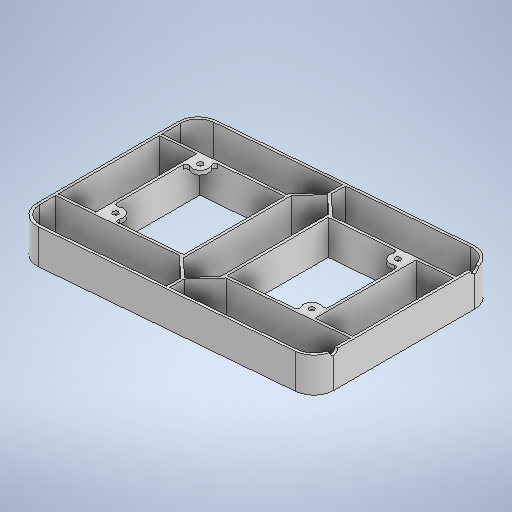
# Autodesk Inventor part: Divider
Saved by Autodesk Inventor 2025.2 (Build 292293000, 293)
## iProperties
Created: 2026-02-06
Part Number: Divider
Material: Generic
Document SubType Name: Modeling
Designer: Joefi
Density: 1 g/cm^3
Appearance: Default
Mass: 74.6343 g
Surface Area: 795.136 cm^2
Volume: 74.6343 cm^3
Author: Joefi
Autodesk Inventor part; units mm, degrees
ref_plane "YZ Plane" through (0, 0, 0) normal (1, 0, 0) x (0, 1, 0)
ref_plane "XZ Plane" through (0, 0, 0) normal (0, 1, 0) x (-1, 0, 0)
ref_plane "XY Plane" through (0, 0, 0) normal (0, 0, 1) x (1, 0, 0)
sketch "Sketch2" plane through (0, 0, 0) normal (0, 1, 0) x (-1, 0, 0)
  line L0 (-103.6195, 45.2048) -> (-103.6195, -60.7112)
  arc A0 (-103.6195, -60.7112) -> (-87.3121, -75.6541) centre (-88.6195, -60.7112) ccw
  line L1 (-87.3121, -75.6541) -> (89.9268, -60.1477)
  arc A1 (89.9268, -60.1477) -> (103.6195, -45.2048) centre (88.6195, -45.2048) ccw
  line L2 (103.6195, -45.2048) -> (103.6195, 60.7112)
  arc A2 (103.6195, 60.7112) -> (87.3121, 75.6541) centre (88.6195, 60.7112) ccw
  line L3 (87.3121, 75.6541) -> (-89.9268, 60.1477)
  arc A3 (-89.9268, 60.1477) -> (-103.6195, 45.2048) centre (-88.6195, 45.2048) ccw
  line L4 (-15, -39.213) -> (-73.7032, -44.3489)
  line L5 (-73.7032, -44.3489) -> (-73.7032, 31.4525)
  line L6 (-73.7032, 31.4525) -> (-15, 36.5884)
  line L7 (-15, 36.5884) -> (-15, -39.213)
  line L8 (73.7032, 44.3489) -> (73.7032, -31.4525)
  line L9 (73.7032, -31.4525) -> (15, -36.5884)
  line L10 (15, -36.5884) -> (15, 39.213)
  line L11 (15, 39.213) -> (73.7032, 44.3489)
  line L12 (-75.7032, -44.5239) -> (-101.6195, -46.7912)
  line L13 (-101.6195, -46.7912) -> (-101.6195, 29.0101)
  line L14 (-101.6195, 29.0101) -> (-75.7032, 31.2775)
  line L15 (-75.7032, 31.2775) -> (-75.7032, -44.5239)
  line L16 (16.0813, -38.5014) -> (101.6195, -31.0178)
  line L17 (101.6195, -31.0178) -> (101.6195, -45.2048)
  arc A4 (89.7525, -58.1553) -> (101.6195, -45.2048) centre (88.6195, -45.2048) ccw
  line L18 (89.7525, -58.1553) -> (1, -65.9202)
  line L19 (1, -65.9202) -> (1, -54.9598)
  line L20 (1, -54.9598) -> (16.0813, -38.5014)
  line L21 (-1, -55.3824) -> (-1, -66.0951)
  line L22 (-1, -66.0951) -> (-87.4864, -73.6617)
  arc A5 (-101.6195, -60.7112) -> (-87.4864, -73.6617) centre (-88.6195, -60.7112) ccw
  line L23 (-101.6195, -60.7112) -> (-101.6195, -48.7989)
  line L24 (-101.6195, -48.7989) -> (-16.3281, -41.3368)
  line L25 (-16.3281, -41.3368) -> (-1, -55.3824)
  line L26 (-16.0813, 38.5014) -> (-101.6195, 31.0178)
  line L27 (-101.6195, 31.0178) -> (-101.6195, 45.2048)
  arc A6 (-89.7525, 58.1553) -> (-101.6195, 45.2048) centre (-88.6195, 45.2048) ccw
  line L28 (-89.7525, 58.1553) -> (-1, 65.9202)
  line L29 (-1, 65.9202) -> (-1, 54.9598)
  line L30 (-1, 54.9598) -> (-16.0813, 38.5014)
  line L31 (13, -39.6468) -> (0.1234, -53.6991)
  line L32 (0.1234, -53.6991) -> (-13, -41.6738)
  line L33 (-13, -41.6738) -> (-13, 39.6468)
  line L34 (-13, 39.6468) -> (-0.1234, 53.6991)
  line L35 (-0.1234, 53.6991) -> (13, 41.6738)
  line L36 (13, 41.6738) -> (13, -39.6468)
  line L37 (101.6195, 46.7912) -> (101.6195, -29.0101)
  line L38 (101.6195, -29.0101) -> (75.7032, -31.2775)
  line L39 (75.7032, -31.2775) -> (75.7032, 44.5239)
  line L40 (75.7032, 44.5239) -> (101.6195, 46.7912)
  line L41 (16.3281, 41.3368) -> (1, 55.3824)
  line L42 (1, 55.3824) -> (1, 66.0951)
  line L43 (1, 66.0951) -> (87.4864, 73.6617)
  arc A7 (101.6195, 60.7112) -> (87.4864, 73.6617) centre (88.6195, 60.7112) ccw
  line L44 (101.6195, 60.7112) -> (101.6195, 48.7989)
  line L45 (101.6195, 48.7989) -> (16.3281, 41.3368)
  point P0 (0, 0)
  point P1 (0, 0)
  constraints: 92 end point, 16 point on circle, 8 centre point
extrude "Extrusion1" add sketch "Sketch2" along normal blind 26
sketch "Sketch3" plane through (0, 0, 0) normal (0, -1, 0) x (1, 0, 0)
  line L0 (-15, 39.213) -> (-73.7032, 44.3489) projected
  line L1 (-73.7032, -31.4525) -> (-15, -36.5884) projected
  line L2 (-73.7032, 44.3489) -> (-73.7032, -31.4525) projected
  line L3 (73.7032, 31.4525) -> (15, 36.5884) projected
  line L4 (73.7032, -44.3489) -> (73.7032, 31.4525) projected
  line L5 (15, -39.213) -> (73.7032, -44.3489) projected
  line L6 (-13.5, 41.8938) -> (0.1542, 54.4056) construction
  line L7 (-0.5, 55.1624) -> (-16.1525, 40.8196) construction
  line L8 (-0.5, 66.5533) -> (-0.5, 55.1624) construction
  line L9 (-15, 39.213) -> (-73.7032, 44.3489) construction
  line L10 (-0.1542, -54.4056) -> (-13.5, -39.8412) construction
  line L11 (-16.1525, 40.8196) -> (-102.1195, 48.3407) construction
  line L12 (-102.1195, 48.3407) -> (-102.1195, 60.7112) construction
  line L13 (16.1525, -40.8196) -> (102.1195, -48.3407) construction
  line L14 (102.1195, 45.2048) -> (102.1195, 30.4721) construction
  line L15 (14.5, 37.134) -> (74.2032, 31.9107) construction
  arc A0 (-87.4429, 74.1598) -> (-102.1195, 60.7112) centre (-88.6195, 60.7112) ccw construction
  line L16 (15.8441, 38.0202) -> (0.5, 54.7653) construction
  line L17 (14.5, -39.6712) -> (14.5, 37.134) construction
  line L18 (13.5, 39.8412) -> (13.5, -41.8938) construction
  line L19 (0.5, -66.5533) -> (0.5, -55.1624) construction
  line L20 (0.5, 66.4658) -> (89.7961, 58.6534) construction
  line L21 (102.1195, 30.4721) -> (15.8441, 38.0202) construction
  line L22 (75.2032, 31.8232) -> (102.1195, 29.4683) construction
  line L23 (74.2032, -44.8945) -> (14.5, -39.6712) construction
  line L24 (0.1542, 54.4056) -> (13.5, 39.8412) construction
  line L25 (13.5, -41.8938) -> (-0.1542, -54.4056) construction
  line L26 (-0.5, -54.7653) -> (-0.5, -66.4658) construction
  line L27 (0.5, 54.7653) -> (0.5, 66.4658) construction
  line L28 (-89.8832, -59.6496) -> (87.3557, -75.156) construction
  line L29 (89.8832, 59.6496) -> (-87.3557, 75.156) construction
  line L30 (-87.4429, 74.1598) -> (-0.5, 66.5533) construction
  arc A1 (-87.3557, 75.156) -> (-103.1195, 60.7112) centre (-88.6195, 60.7112) ccw construction
  line L31 (87.4429, -74.1598) -> (0.5, -66.5533) construction
  line L32 (74.2032, 31.9107) -> (74.2032, -44.8945) construction
  line L33 (75.2032, -44.982) -> (75.2032, 31.8232) construction
  line L34 (102.1195, 29.4683) -> (102.1195, -47.3369) construction
  line L35 (102.1195, -48.3407) -> (102.1195, -60.7112) construction
  line L36 (103.1195, -60.7112) -> (103.1195, 45.2048) construction
  arc A2 (-102.1195, -45.2048) -> (-89.7961, -58.6534) centre (-88.6195, -45.2048) ccw construction
  arc A3 (-103.1195, -45.2048) -> (-89.8832, -59.6496) centre (-88.6195, -45.2048) ccw construction
  line L37 (0.5, -55.1624) -> (16.1525, -40.8196) construction
  arc A4 (102.1195, 45.2048) -> (89.7961, 58.6534) centre (88.6195, 45.2048) ccw construction
  arc A5 (103.1195, 45.2048) -> (89.8832, 59.6496) centre (88.6195, 45.2048) ccw construction
  line L38 (-15.8441, -38.0202) -> (-0.5, -54.7653) construction
  line L39 (-0.5, -66.4658) -> (-89.7961, -58.6534) construction
  line L40 (-13.5, -39.8412) -> (-13.5, 41.8938) construction
  line L41 (-15, -36.5884) -> (-15, 39.213) construction
  line L42 (-102.1195, 47.3369) -> (-75.2032, 44.982) construction
  line L43 (-75.2032, 44.982) -> (-75.2032, -31.8232) construction
  line L44 (-73.7032, 44.3489) -> (-73.7032, -31.4525) construction
  line L45 (-102.1195, -29.4683) -> (-102.1195, 47.3369) construction
  line L46 (-75.2032, -31.8232) -> (-102.1195, -29.4683) construction
  line L47 (-103.1195, 60.7112) -> (-103.1195, -45.2048) construction
  line L48 (-73.7032, -31.4525) -> (-15, -36.5884) construction
  line L49 (-102.1195, -45.2048) -> (-102.1195, -30.4721) construction
  line L50 (-102.1195, -30.4721) -> (-15.8441, -38.0202) construction
  line L51 (102.1195, -47.3369) -> (75.2032, -44.982) construction
  arc A6 (87.4429, -74.1598) -> (102.1195, -60.7112) centre (88.6195, -60.7112) ccw construction
  arc A7 (87.3557, -75.156) -> (103.1195, -60.7112) centre (88.6195, -60.7112) ccw construction
  circle A8 centre (-67.7032, -25.9545) radius 6
  circle A9 centre (-67.7032, 37.801) radius 6
  circle A10 centre (68.2032, -38.3467) radius 6
  circle A11 centre (68.2032, 26.4127) radius 6
  circle A12 centre (-67.7032, -25.9545) radius 1.45 construction
  circle A13 centre (-67.7032, 37.801) radius 1.45 construction
  circle A14 centre (68.2032, 26.4127) radius 1.45 construction
  circle A15 centre (68.2032, -38.3467) radius 1.45 construction
  line L52 (-100.0356, -54.4397) -> (-99.164, -44.4778)
  line L53 (-99.164, -44.4778) -> (-95.4115, -44.8061)
  line L54 (-95.4115, -44.8061) -> (-95.4115, 61.1557)
  line L55 (-95.4115, 61.1557) -> (-100.0356, 61.5603)
  line L56 (-100.0356, 61.5603) -> (-99.164, 71.5222)
  line L57 (-99.164, 71.5222) -> (96.0902, 54.4397)
  line L58 (96.0902, 54.4397) -> (95.2186, 44.4778)
  line L59 (95.2186, 44.4778) -> (91.4661, 44.8061)
  line L60 (91.4661, 44.8061) -> (91.4661, -61.1557)
  line L61 (91.4661, -61.1557) -> (96.0902, -61.5603)
  line L62 (96.0902, -61.5603) -> (95.2186, -71.5222)
  line L63 (95.2186, -71.5222) -> (-100.0356, -54.4397)
  arc A16 (-119, 83.3333) -> (-125, 77.3333) centre (-119, 77.3333) ccw
  line L64 (-125, 77.3333) -> (-125, -77.3333)
  arc A17 (-125, -77.3333) -> (-119, -83.3333) centre (-119, -77.3333) ccw
  line L65 (-119, -83.3333) -> (119, -83.3333)
  arc A18 (119, -83.3333) -> (125, -77.3333) centre (119, -77.3333) ccw
  line L66 (125, -77.3333) -> (125, 77.3333)
  arc A19 (125, 77.3333) -> (119, 83.3333) centre (119, 77.3333) ccw
  line L67 (119, 83.3333) -> (-119, 83.3333)
  circle A20 centre (119, -77.3333) radius 2
  circle A21 centre (119, 77.3333) radius 2
  circle A22 centre (-119, 77.3333) radius 2
  circle A23 centre (-119, -77.3333) radius 2
  circle A24 centre (68.2032, 26.4127) radius 2
  circle A25 centre (68.2032, -38.3467) radius 2
  circle A26 centre (-67.7032, -25.9545) radius 2
  circle A27 centre (-67.7032, 37.801) radius 2
  point P0 (0, 0)
  point P1 (0, 0)
  point P2 (0, 0)
  point P3 (0, 0)
  point P4 (88.6195, -7.7532)
  point P5 (-88.6195, 7.7532)
  point P6 (-68.2261, -31.9317)
  point P7 (-73.7032, -25.9545)
  point P8 (-73.7032, 37.801)
  point P9 (-67.1803, 43.7782)
  point P10 (73.7032, -35.9488)
  point P11 (65.335, -43.6168)
  point P12 (66.2938, 32.1007)
  point P13 (73.7032, 24.0148)
  dimension "d2" = 12
  dimension "d3" = 12
  dimension "d4" = 12
  dimension "d5" = 12
  dimension "d6" = 2.9
  dimension "d16" = 4
  dimension "d17" = 4
  dimension "d18" = 4
  dimension "d19" = 4
  constraints: 124 end point, 28 centre point, 24 point on circle, 8 coincident, 8 tangent, 3 equal radius
  measures "d2" diameter of A8
  measures "d3" diameter of A9
  measures "d4" diameter of A10
  measures "d5" diameter of A11
  measures "d6" diameter of A12
  measures "d16" diameter of A24
  measures "d17" diameter of A25
  measures "d18" diameter of A26
  measures "d19" diameter of A27
extrude "Extrusion2" add sketch "Sketch3" along normal blind 3 from surface at -26 contours A9 L2 L0 | A9 | L2 A8 L1 | A8 | L4 A11 L3 | A11 L4 L3 | L5 A10 L4 | A10 L5 L4
fillet "Fillet1" radius 2 8 edges at (-68.2261, 24.5, -31.9317) (-73.7032, 24.5, -25.9545) (-73.7032, 24.5, 37.801) (-67.1803, 24.5, 43.7782) (73.7032, 24.5, 24.0148) (66.2938, 24.5, 32.1007) (73.7032, 24.5, -35.9488) (65.335, 24.5, -43.6168)
chamfer "Chamfer1" distance 1 angle 45 4 edges at (-69.7032, 23, -25.9545) (-69.7032, 23, 37.801) (66.2032, 23, 26.4127) (66.2032, 23, -38.3467)
sketch "Sketch6" plane through (103.6195, 0, 45.2048) normal (1, 0, 0) x (0, 0, -1)
  circle A0 centre (0, 26) radius 3
  circle A1 centre (105.916, 26) radius 3
  point P0 (45.2048, 0)
  dimension "d23" = 6
  dimension "d26" = 6
  constraints: 2 centre point, 2 coincident
  measures "d23" diameter of A0
  measures "d26" diameter of A1
extrude "Extrusion4" cut sketch "Sketch6" against normal blind 27
body "Solid1"
